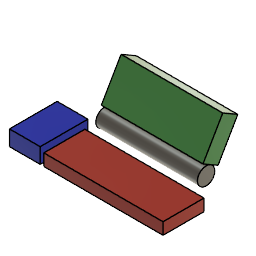
Rough+Cyberdeck+2 (Autodesk Fusion 360 design; units mm, degrees)
part number: 2025-05-15-11-44-52-619
Autodesk Fusion 360 part; units mm, degrees
sketch "Sketch1" plane through (0, 0, 0) normal (0, 0, 1) x (1, 0, 0)
  line L0 (-116, 40) -> (116, 40)
  line L1 (116, 40) -> (116, -40)
  line L2 (116, -40) -> (-116, -40)
  line L3 (-116, -40) -> (-116, 40)
  line L4 (-116, 40) -> (116, -40) construction
  line L5 (116, 40) -> (-116, -40) construction
  dimension "d1" = 80
  dimension "d2" = 232
  constraint horizontal L0
  constraint perpendicular L0 L1
  constraint parallel L0 L2
  constraint parallel L1 L3
  constraint coincident L4 origin
  constraint coincident L5 origin
  measures "d1" distance of L0.start L2.end
  measures "d2" distance of L0.start L0.end
extrude "Extrude1" add sketch "Sketch1" along normal blind 23 makes body 1
sketch "Sketch2" plane through (0, 0, 23) normal (0, 0, 1) x (-1, 0, 0)
  line L0 (116, 40) -> (-116, 40)
  line L1 (-116, 40) -> (-116, -40)
  line L2 (-116, -40) -> (116, -40)
  line L3 (116, -40) -> (116, 40)
  line L4 (96.6813, -126.5449) -> (-101.3187, -126.5449)
  line L5 (-101.3187, -126.5449) -> (-101.3187, -203.5449)
  line L6 (-101.3187, -203.5449) -> (96.6813, -203.5449)
  line L7 (96.6813, -203.5449) -> (96.6813, -126.5449)
  line L8 (96.6813, -126.5449) -> (-101.3187, -203.5449) construction
  line L9 (-101.3187, -126.5449) -> (96.6813, -203.5449) construction
  point P0 (-2.3187, -165.0449)
  dimension "d5" = 198
  dimension "d6" = 77
  constraint horizontal L4
  constraint perpendicular L4 L5
  constraint parallel L4 L6
  constraint parallel L5 L7
  constraint coincident L8 P0
  constraint coincident L9 P0
  measures "d5" distance of L4.start L4.end
  measures "d6" distance of L4.end L5.end
extrude "Extrude2" add sketch "Sketch2" along normal blind 34 separate body contours L4 L5 L6 L7 makes body 2
sketch "Sketch3" plane through (0, 0, 0) normal (0, 0, 1) x (1, 0, 0)
  line L0 (323, 30) -> (230, 30)
  line L1 (230, 30) -> (230, -30)
  line L2 (230, -30) -> (323, -30)
  line L3 (323, -30) -> (323, 30)
  line L4 (323, 30) -> (230, -30) construction
  line L5 (230, 30) -> (323, -30) construction
  point P0 (276.5, 0)
  dimension "d9" = 60
  dimension "d10" = 93
  constraint horizontal L0
  constraint perpendicular L0 L1
  constraint parallel L0 L2
  constraint parallel L1 L3
  constraint coincident L4 P0
  constraint coincident L5 P0
  measures "d9" distance of L0.end L1.end
  measures "d10" distance of L0.start L0.end
extrude "Extrude3" add sketch "Sketch3" along normal blind 30 separate body makes body 3
move_body "Move1" bodies 2 to x (1, 0, 0) y (0, 0.5, 0.866025) z (0, -0.866025, 0.5) at (0, 128.1213, -107.9126)
move_body "Move2" bodies 2 to x (1, 0, 0) y (0, 1, 0) z (0, 0, 1) at (-2.3187, -102.0303, -7.1786)
move_body "Move3" bodies 2 to x (1, 0, 0) y (0, 1, 0) z (0, 0, 1) at (0, 10, 0)
move_body "Move4" bodies 3 to x (1, 0, 0) y (0, 1, 0) z (0, 0, 1) at (-275, 125, 0)
move_body "Move5" bodies 3 to x (1, 0, 0) y (0, 1, 0) z (0, 0, 1) at (0, 3, 0)
move_body "Move6" bodies 3 to x (1, 0, 0) y (0, 1, 0) z (0, 0, 1) at (-1.5, -18.5551, 6)
move_body "Move7" bodies 3 to x (1, 0, 0) y (0, 1, 0) z (0, 0, 1) at (0, 24, 0)
move_body "Move8" bodies 3 to x (1, 0, 0) y (0, 1, 0) z (0, 0, 1) at (0, -63.4449, -6)
move_body "Move9" bodies 3 to x (1, 0, 0) y (0, 1, 0) z (0, 0, 1) at (0, 60, 0)
move_body "Move10" bodies 2 to x (1, 0, 0) y (0, 1, 0) z (0, 0, 1) at (0, 0, 60)
move_body "Move11" bodies 3 to x (1, 0, 0) y (0, 1, 0) z (0, 0, 1) at (0, -50, 0)
move_body "Move12" bodies 2 to x (1, 0, 0) y (0, 1, 0) z (0, 0, 1) at (0, -5, -25)
move_body "Move13" bodies 3 to x (1, 0, 0) y (0, 1, 0) z (0, 0, 1) at (0, 65, 0)
move_body "Move14" bodies 2 to x (1, 0, 0) y (0, 0.866025, 0.5) z (0, -0.5, 0.866025) at (0, 26.5289, -17.007)
move_body "Move15" bodies 3 to x (0, 1, 0) y (-1, 0, 0) z (0, 0, 1) at (-3, 6.5, 0)
move_body "Move16" bodies 3 to x (1, 0, 0) y (0, 1, 0) z (0, 0, 1) at (-5, 0, 0)
sketch "Sketch4" plane through (0, 0, 23) normal (0, 0, 1) x (1, 0, 0)
move_body "Move17" bodies 2 to x (1, 0, 0) y (0, 1, 0) z (0, 0, 1) at (0, 30, 0)
sketch "Sketch5" plane through (99, 0, 0) normal (1, 0, 0) x (0, 1, 0)
  line L0 (100.5, 55.7224) -> (100.5, 132.7224)
  line L1 (100.5, 132.7224) -> (66.5, 132.7224)
  line L2 (66.5, 132.7224) -> (66.5, 55.7224)
  line L3 (66.5, 55.7224) -> (100.5, 55.7224) construction
  line L4 (66.5, 55.7224) -> (100.5, 55.7224) construction
  line L5 (100.5, 55.7224) -> (100.5, 21.7224) construction
  line L6 (100.5, 21.7224) -> (66.5, 21.7224) construction
  line L7 (66.5, 21.7224) -> (66.5, 55.7224) construction
  circle A0 centre (83.5, 38.7224) radius 17
  dimension "d34" = 34
  dimension "d35" = 34
  constraint horizontal L4
  constraint vertical L5
  constraint horizontal L6
  constraint vertical L7
  constraint coincident L2.end L3.start
  constraint tangent L5 A0
  measures "d34" distance of L2.end L6.end
  measures "d35" distance of L2.end L0.start
extrude "Extrude4" add sketch "Sketch5" against normal up to surface (198 mm away) separate body makes body 4
move_body "Move18" bodies 4 2 to x (1, 0, 0) y (0, 0, 1) z (0, -1, 0) at (0, 99.7224, -42.2776)
move_body "Move19" bodies 2 4 to x (1, 0, 0) y (0, -0.5, -0.866025) z (0, 0.866025, -0.5) at (0, 55.8003, 114.6612)
